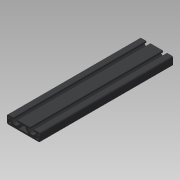
# Autodesk Inventor part: 3075
Saved by Autodesk Inventor 2013 (Build 170138000, 138)
## iProperties
Company: 80/20 Inc.
Created: 2014-04-23
Part Number: 3075
Material: Generic
Document SubType Name: Modeling
Density: 1 g/cm^3
Vendor: 80/20 Inc.
Engineer: Ross Bowman
Designer: Ross Bowman
Catalog Web Link: 8020.net
Material: 6105-T5 Aluminum
Author: Ross Bowman
Keywords: 80/20 , 8020 , T-Slot , Extrusion
Autodesk Inventor part; units mm, degrees
ref_plane "YZ Plane" through (0, 0, 0) normal (1, 0, 0) x (0, 1, 0)
ref_plane "XZ Plane" through (0, 0, 0) normal (0, 1, 0) x (-1, 0, 0)
ref_plane "XY Plane" through (0, 0, 0) normal (0, 0, 1) x (1, 0, 0)
sketch "Sketch1" plane through (0, 0, 0) normal (0, 0, 1) x (1, 0, 0)
  circle A0 centre (31.75, -3.175) radius 3.3274
  circle A1 centre (33.8988, 5.2764) radius 2.5527
  circle A2 centre (-33.8988, 5.2764) radius 2.5527
  circle A3 centre (-31.75, -3.175) radius 3.3274
  line L0 (-9.5899, -5.461) -> (9.5899, -5.461)
  arc A4 (-10.4789, -4.572) -> (-9.5899, -5.461) centre (-9.5899, -4.572) ccw
  line L1 (-10.4789, -4.1197) -> (-10.4789, -4.572)
  arc A5 (-10.2185, -3.4911) -> (-10.4789, -4.1197) centre (-9.5899, -4.1197) ccw
  line L2 (-6.264, 0.4634) -> (-10.2185, -3.4911)
  arc A6 (-6.264, 0.4634) -> (-4.8728, 3.822) centre (-9.6226, 3.822) ccw
  line L3 (-4.8728, 4.191) -> (-4.8728, 3.822)
  arc A7 (-3.6028, 5.461) -> (-4.8728, 4.191) centre (-3.6028, 4.191) ccw
  line L4 (3.6028, 5.461) -> (-3.6028, 5.461)
  arc A8 (4.8728, 4.191) -> (3.6028, 5.461) centre (3.6028, 4.191) ccw
  line L5 (4.8728, 3.822) -> (4.8728, 4.191)
  arc A9 (4.8728, 3.822) -> (6.264, 0.4634) centre (9.6226, 3.822) ccw
  line L6 (10.2185, -3.4911) -> (6.264, 0.4634)
  arc A10 (10.4789, -4.1197) -> (10.2185, -3.4911) centre (9.5899, -4.1197) ccw
  line L7 (10.4789, -4.572) -> (10.4789, -4.1197)
  arc A11 (9.5899, -5.461) -> (10.4789, -4.572) centre (9.5899, -4.572) ccw
  arc A12 (24.638, 9.525) -> (23.114, 8.001) centre (24.638, 8.001) ccw
  line L8 (23.114, 8.001) -> (23.114, 6.731)
  arc A13 (23.114, 6.731) -> (24.384, 5.461) centre (24.384, 6.731) ccw
  line L9 (24.384, 5.461) -> (28.448, 5.461)
  arc A14 (29.337, 4.572) -> (28.448, 5.461) centre (28.448, 4.572) ccw
  line L10 (29.337, 4.572) -> (29.337, 4.2554)
  arc A15 (29.0766, 3.6267) -> (29.337, 4.2554) centre (28.448, 4.2554) ccw
  line L11 (29.0766, 3.6267) -> (24.1741, -1.2758)
  arc A16 (20.8154, -2.667) -> (24.1741, -1.2758) centre (20.8154, 2.0828) ccw
  line L12 (20.8154, -2.667) -> (17.2846, -2.667)
  arc A17 (13.9259, -1.2758) -> (17.2846, -2.667) centre (17.2846, 2.0828) ccw
  line L13 (13.9259, -1.2758) -> (9.0234, 3.6267)
  arc A18 (8.763, 4.2554) -> (9.0234, 3.6267) centre (9.652, 4.2554) ccw
  line L14 (8.763, 4.2554) -> (8.763, 4.572)
  arc A19 (9.652, 5.461) -> (8.763, 4.572) centre (9.652, 4.572) ccw
  line L15 (9.652, 5.461) -> (13.716, 5.461)
  arc A20 (13.716, 5.461) -> (14.986, 6.731) centre (13.716, 6.731) ccw
  line L16 (14.986, 6.731) -> (14.986, 8.001)
  arc A21 (14.986, 8.001) -> (13.462, 9.525) centre (13.462, 8.001) ccw
  line L17 (13.462, 9.525) -> (-13.462, 9.525)
  arc A22 (-13.462, 9.525) -> (-14.986, 8.001) centre (-13.462, 8.001) ccw
  line L18 (-14.986, 8.001) -> (-14.986, 6.731)
  arc A23 (-14.986, 6.731) -> (-13.716, 5.461) centre (-13.716, 6.731) ccw
  line L19 (-13.716, 5.461) -> (-9.652, 5.461)
  arc A24 (-8.763, 4.572) -> (-9.652, 5.461) centre (-9.652, 4.572) ccw
  line L20 (-8.763, 4.572) -> (-8.763, 4.2554)
  arc A25 (-9.0234, 3.6267) -> (-8.763, 4.2554) centre (-9.652, 4.2554) ccw
  line L21 (-9.0234, 3.6267) -> (-13.9259, -1.2758)
  arc A26 (-17.2846, -2.667) -> (-13.9259, -1.2758) centre (-17.2846, 2.0828) ccw
  line L22 (-17.2846, -2.667) -> (-20.8154, -2.667)
  arc A27 (-24.1741, -1.2758) -> (-20.8154, -2.667) centre (-20.8154, 2.0828) ccw
  line L23 (-24.1741, -1.2758) -> (-29.0766, 3.6267)
  arc A28 (-29.337, 4.2554) -> (-29.0766, 3.6267) centre (-28.448, 4.2554) ccw
  line L24 (-29.337, 4.2554) -> (-29.337, 4.572)
  arc A29 (-28.448, 5.461) -> (-29.337, 4.572) centre (-28.448, 4.572) ccw
  line L25 (-28.448, 5.461) -> (-24.384, 5.461)
  arc A30 (-24.384, 5.461) -> (-23.114, 6.731) centre (-24.384, 6.731) ccw
  line L26 (-23.114, 6.731) -> (-23.114, 8.001)
  arc A31 (-23.114, 8.001) -> (-24.638, 9.525) centre (-24.638, 8.001) ccw
  line L27 (-24.638, 9.525) -> (-34.925, 9.525)
  arc A32 (-34.925, 9.525) -> (-38.1, 6.35) centre (-34.925, 6.35) ccw
  line L28 (-38.1, 6.35) -> (-38.1, -6.35)
  arc A33 (-38.1, -6.35) -> (-34.925, -9.525) centre (-34.925, -6.35) ccw
  line L29 (-34.925, -9.525) -> (34.925, -9.525)
  arc A34 (34.925, -9.525) -> (38.1, -6.35) centre (34.925, -6.35) ccw
  line L30 (38.1, -6.35) -> (38.1, 6.35)
  arc A35 (38.1, 6.35) -> (34.925, 9.525) centre (34.925, 6.35) ccw
  line L31 (34.925, 9.525) -> (24.638, 9.525)
  point P0 (0, 0)
  constraints: 64 end point, 64 point on circle, 36 centre point
extrude "Extrusion1" add sketch "Sketch1" against normal blind 304.8
body "Solid1"
